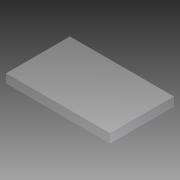
# Autodesk Inventor part: Window
Saved by Autodesk Inventor 2011 SP2 (Build 150309200, 309)
## iProperties
Created: 2012-03-02
Part Number: Window
Document SubType Name: Modeling
Designer: sungwook
Density: 1 g/cm^3
Author: sungwook
Autodesk Inventor part; units mm, degrees
ref_plane "YZ Plane" through (0, 0, 0) normal (1, 0, 0) x (0, 1, 0)
ref_plane "XZ Plane" through (0, 0, 0) normal (0, 1, 0) x (-1, 0, 0)
ref_plane "XY Plane" through (0, 0, 0) normal (0, 0, 1) x (1, 0, 0)
sketch "Sketch1" plane through (0, 0, 0) normal (0, 0, 1) x (1, 0, 0)
  line L0 (-17.5, 10.75) -> (17.5, 10.75)
  line L1 (17.5, 10.75) -> (17.5, -10.75)
  line L2 (17.5, -10.75) -> (-17.5, -10.75)
  line L3 (-17.5, -10.75) -> (-17.5, 10.75)
  point P0 (0, 0)
  point P1 (0, 10.75)
  point P2 (-17.5, 0)
  dimension "d0" = 35
  dimension "d1" = 21.5
  constraints: 8 end point, 2 midpoint, 2 parallel, 1 horizontal, 1 horizontal alignment, 1 perpendicular, 1 vertical alignment
  measures "d0" distance between parallel lines of L1 L3
  measures "d1" distance of L2.end L0.start
extrude "Extrusion1" add sketch "Sketch1" along normal blind 3
body "Solid1"
